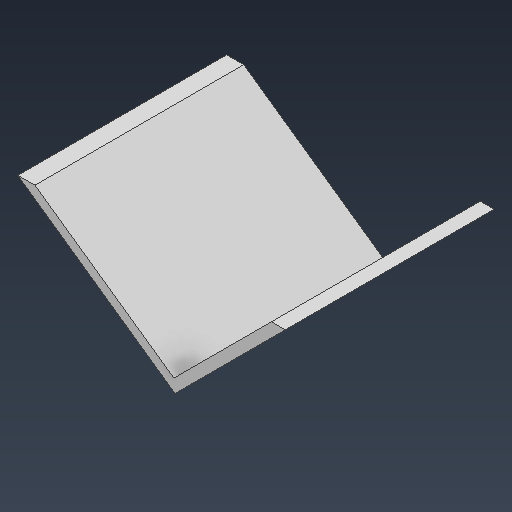
# Autodesk Inventor part: ХУЙ
Saved by Autodesk Inventor 2026 (Build 300175000, 175)
## iProperties
Created: 2026-01-11
Part Number: ХУЙ
Material: Типовые
Document SubType Name: Modeling
Designer: GameHD
Density: 1 g/cm^3
Appearance: По умолчанию
Author: GameHD
Autodesk Inventor part; units mm, degrees
ref_plane "YZ Plane" through (0, 0, 0) normal (1, 0, 0) x (0, 1, 0)
ref_plane "XZ Plane" through (0, 0, 0) normal (0, 1, 0) x (-1, 0, 0)
ref_plane "XY Plane" through (0, 0, 0) normal (0, 0, 1) x (1, 0, 0)
sketch "Эскиз1" plane through (0, 0, 0) normal (0, 0, 1) x (1, 0, 0)
  line L0 (0, 0) -> (120, 0)
  line L1 (120, 0) -> (70.5025, -49.4975)
  line L2 (70.5025, -49.4975) -> (0, 0)
  line L3 (-12.6589, 4) -> (129.6569, 4)
  line L4 (129.6569, 4) -> (70.9546, -54.7022)
  line L5 (70.9546, -54.7022) -> (-12.6589, 4)
  line L6 (6.9888, -9.794) -> (115.8629, -9.794)
  point P0 (110.206, -9.794)
  point P1 (13.9502, -9.794)
  dimension "d0" = 120
  dimension "d1" = 70
  dimension "d2" = 45
  dimension "d3" = 4
  constraints: 14 end point, 2 horizontal, 2 point on line, 2 other
  measures "d0" distance of L0.start L0.end
  measures "d1" distance of L0.end L1.end
  measures "d2" angle of L0 L1
  measures "d3" distance between parallel lines of L2 L5
extrude "Выдавливание1" add sketch "Эскиз1" along normal blind 85 contours L2 L1 L6 L4 L5
